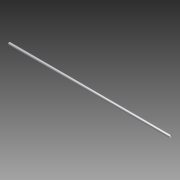
# Autodesk Inventor part: rod-long
Saved by Autodesk Inventor 2013 (Build 170138000, 138)
## iProperties
Created: 2013-09-24
Part Number: rod-long
Material: Aluminum 6061
Document SubType Name: Modeling
Designer: Admin
Mass: 72.6299 g
Surface Area: 658.298 cm^2
Volume: 26.8007 cm^3
Density: 2.71 g/cm^3
Author: Admin
Autodesk Inventor part; units mm, degrees
ref_plane "YZ Plane" through (0, 0, 0) normal (1, 0, 0) x (0, 1, 0)
ref_plane "XZ Plane" through (0, 0, 0) normal (0, 1, 0) x (-1, 0, 0)
ref_plane "XY Plane" through (0, 0, 0) normal (0, 0, 1) x (1, 0, 0)
sketch "Sketch1" plane through (0, 0, 0) normal (1, 0, 0) x (0, 1, 0)
  circle A0 centre (0, 0) radius 6.38
  circle A1 centre (0, 0) radius 5.565
  dimension "d0" = 12.76
  dimension "d1" = 11.13
  constraints: 2 centre point, 1 coincident
  measures "d0" diameter of A0
  measures "d1" diameter of A1
extrude "Extrusion1" add sketch "Sketch1" along normal blind 876.3
body "Solid1"
